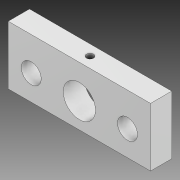
# Autodesk Inventor part: 1234_Spool Plate_V1
Saved by Autodesk Inventor 2020 (Build 240168000, 168)
## iProperties
Created: 2019-09-27
Part Number: 1234_Spool Plate_V1
Material: Aluminum
Document SubType Name: Modeling
Designer: MPI
Density: 2.7 g/cm^3
Appearance: Satin
Author: MPI
Autodesk Inventor part; units mm, degrees
ref_plane "YZ Plane" through (0, 0, 0) normal (1, 0, 0) x (0, 1, 0)
ref_plane "XZ Plane" through (0, 0, 0) normal (0, 1, 0) x (-1, 0, 0)
ref_plane "XY Plane" through (0, 0, 0) normal (0, 0, 1) x (1, 0, 0)
sketch "Sketch1" plane through (0, 0, 0) normal (0, 0, 1) x (1, 0, 0)
  circle A0 centre (0, 0) radius 19.25
  line L0 (-85, 40) -> (85, 40)
  line L1 (85, 40) -> (85, -30)
  line L2 (85, -30) -> (-85, -30)
  line L3 (-85, -30) -> (-85, 40)
  circle A1 centre (57.5, 0) radius 11.905
  circle A2 centre (-57.5, 0) radius 11.905
  dimension "d0" = 38.5
  dimension "d1" = 23.81
  dimension "d2" = 23.81
  dimension "d3" = 57.5
  dimension "d4" = 57.5
  dimension "d5" = 170
  dimension "d6" = 85
  dimension "d7" = 70
  dimension "d8" = 40
  constraints: 8 end point, 3 centre point, 2 parallel, 1 coincident, 1 horizontal, 1 perpendicular
  measures "d0" diameter of A0
  measures "d1" diameter of A1
  measures "d2" diameter of A2
  measures "d3" distance of A2.centre point (0, 0)
  measures "d4" distance of A1.centre point (0, 0)
  measures "d5" distance of L0.start L0.end
  measures "d6" distance from line of point (0, 0) L3
  measures "d7" distance of L0.end L1.end
  measures "d8" distance from line of point (0, 0) L0
extrude "Extrusion1" add sketch "Sketch1" along normal blind 25.4
sketch "Sketch2" plane through (-85, 40, 0) normal (0, 1, 0) x (1, 0, 0)
  circle A0 centre (85, -12.7) radius 4.215
  line L0 (170, 0) -> (170, -25.4) projected
  point P0 (85, 0)
  dimension "d11" = 8.43
  dimension "d12" = 12.7
  dimension "d13" = 85
  constraints: 1 centre point
  measures "d11" diameter of A0
  measures "d12" distance of A0.centre point (85, 0)
  measures "d13" distance from line of L0 A0.centre
extrude "Extrusion2" cut sketch "Sketch2" against normal blind 25.4
body "Solid1"
